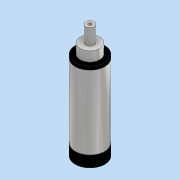
# Autodesk Inventor part: Wrzeciono Elektrowrzeciono CNC 0.8kw
Saved by Autodesk Inventor 2018 (Build 220112000, 112)
## iProperties
Created: 2019-01-26
Part Number: Wrzeciono Elektrowrzeciono CNC 0.8kw
Material: Ogólny
Document SubType Name: Modeling
Designer: Dawid
Density: 1 g/cm^3
Appearance: Domyślna
Author: Dawid
Autodesk Inventor part; units mm, degrees
ref_plane "YZ Plane" through (0, 0, 0) normal (1, 0, 0) x (0, 1, 0)
ref_plane "XZ Plane" through (0, 0, 0) normal (0, 1, 0) x (-1, 0, 0)
ref_plane "XY Plane" through (0, 0, 0) normal (0, 0, 1) x (1, 0, 0)
sketch "Szkic1" plane through (0, 0, 0) normal (0, 0, 1) x (1, 0, 0)
  circle A0 centre (0, 0) radius 32.5
  dimension "d0" = 65
  constraints: 1 centre point, 1 coincident
  measures "d0" diameter of A0
extrude "Wyciągnięcie proste1" add sketch "Szkic1" along normal blind 164
sketch "Szkic2" plane through (0, 0, 0) normal (0, 0, -1) x (-1, 0, 0)
  circle A0 centre (0, 0) radius 32.5 projected
  circle A1 centre (0, 0) radius 33
  dimension "d3" = 66
  constraints: 1 centre point, 1 coincident
  measures "d3" diameter of A1
extrude "Wyciągnięcie proste2" add sketch "Szkic2" along normal blind 25 contours A0 | A1
sketch "Szkic3" plane through (0, 0, 164) normal (0, 0, 1) x (1, 0, 0)
  circle A0 centre (0, 0) radius 33
  dimension "d6" = 66
  constraints: 1 centre point, 1 coincident
  measures "d6" diameter of A0
extrude "Wyciągnięcie proste3" add sketch "Szkic3" along normal blind 8
sketch "Szkic4" plane through (0, 0, 172) normal (0, 0, 1) x (1, 0, 0)
  circle A0 centre (0, 0) radius 22
  dimension "d9" = 44
  constraints: 1 centre point, 1 coincident
  measures "d9" diameter of A0
extrude "Wyciągnięcie proste4" add sketch "Szkic4" along normal blind 22
sketch "Szkic5" plane through (0, 0, 194) normal (0, 0, 1) x (1, 0, 0)
  circle A0 centre (0, 0) radius 9.5
  dimension "d12" = 19
  constraints: 1 centre point, 1 coincident
  measures "d12" diameter of A0
extrude "Wyciągnięcie proste5" add sketch "Szkic5" along normal blind 36
sketch "Szkic6" plane through (0, 0, 230) normal (0, 0, 1) x (1, 0, 0)
  circle A0 centre (0, 0) radius 4
  dimension "d15" = 8
  constraints: 1 centre point, 1 coincident
  measures "d15" diameter of A0
extrude "Wyciągnięcie proste6" cut sketch "Szkic6" against normal blind 30
